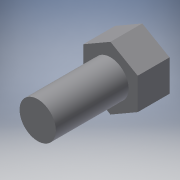
# Autodesk Inventor part: short half-inch hex bolt
Saved by Autodesk Inventor 2016 (Build 200138000, 138)
## iProperties
Created: 2016-01-17
Part Number: short half-inch hex bolt
Material: Steel
Document SubType Name: Modeling
Designer: gus
Density: 7.85 g/cm^3
Appearance: Plate
Author: gus
Autodesk Inventor part; units mm, degrees
ref_plane "YZ Plane" through (0, 0, 0) normal (1, 0, 0) x (0, 1, 0)
ref_plane "XZ Plane" through (0, 0, 0) normal (0, 1, 0) x (-1, 0, 0)
ref_plane "XY Plane" through (0, 0, 0) normal (0, 0, 1) x (1, 0, 0)
sketch "Sketch1" plane through (0, 0, 0) normal (0, 0, 1) x (1, 0, 0)
  line L0 (-9.525, 5.4993) -> (0, 10.9985)
  line L1 (0, 10.9985) -> (9.525, 5.4993)
  line L2 (9.525, 5.4993) -> (9.525, -5.4993)
  line L3 (9.525, -5.4993) -> (0, -10.9985)
  line L4 (0, -10.9985) -> (-9.525, -5.4993)
  line L5 (-9.525, -5.4993) -> (-9.525, 5.4993)
  point P0 (0, 0)
  point P1 (0, 0)
  dimension "d0" = 19.05
  constraints: 12 end point, 1 coincident, 1 vertical, 13 other
  measures "d0" distance between parallel lines of L2 L5
extrude "Extrusion1" add sketch "Sketch1" along normal blind 11.1125
sketch "Sketch2" plane through (0, 0, 11.1125) normal (0, 0, 1) x (1, 0, 0)
  circle A0 centre (0, 0) radius 6.35
  point P0 (0, 0)
  dimension "d3" = 12.7
  constraints: 1 centre point, 1 coincident
  measures "d3" diameter of A0
extrude "Extrusion2" add sketch "Sketch2" along normal blind 25.4
body "Solid1"
